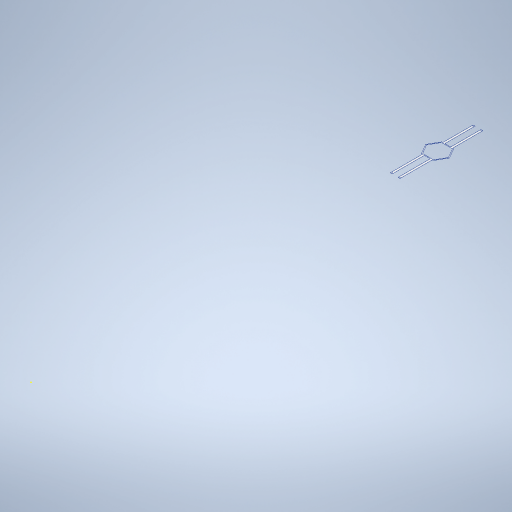
# Autodesk Inventor part: Suporte Drone
Saved by Autodesk Inventor 2024 (Build 280153000, 153)
## iProperties
Created: 2024-05-05
Part Number: Suporte Drone
Material: Alumínio 6061
Document SubType Name: Modeling
Designer: mathe
Density: 2.7 g/cm^3
Appearance: Alumínio - Plano
Author: mathe
Autodesk Inventor part; units mm, degrees
ref_plane "YZ Plane" through (0, 0, 0) normal (1, 0, 0) x (0, 1, 0)
ref_plane "XZ Plane" through (0, 0, 0) normal (0, 1, 0) x (-1, 0, 0)
ref_plane "XY Plane" through (0, 0, 0) normal (0, 0, 1) x (1, 0, 0)
sketch "Esboço1" plane through (0, 0, 0) normal (0, 1, 0) x (-1, 0, 0)
  circle A0 centre (4056.1731, -3688.1035) radius 2.5
  circle A1 centre (4056.1731, -4511.1035) radius 2.5
  circle A2 centre (3976.1731, -3688.1035) radius 2.5
  circle A3 centre (3976.1731, -4511.1035) radius 2.5
  line L0 (3904.5296, -4109.6035) -> (3960.3514, -4012.9174)
  line L1 (3960.3514, -4012.9174) -> (4071.9948, -4012.9174)
  line L2 (4071.9948, -4012.9174) -> (4127.8165, -4109.6035)
  line L3 (4127.8165, -4109.6035) -> (4071.9948, -4206.2895)
  line L4 (4071.9948, -4206.2895) -> (3960.3514, -4206.2895)
  line L5 (3960.3514, -4206.2895) -> (3904.5296, -4109.6035)
  line L6 (4136.5404, -4109.6035) -> (4076.3567, -4213.8446)
  line L7 (3955.9894, -4213.8446) -> (3895.8058, -4109.6035)
  line L8 (3895.8058, -4109.6035) -> (3955.9894, -4005.3623)
  line L9 (4076.3567, -4005.3623) -> (4136.5404, -4109.6035)
  line L10 (3986.1731, -3678.1035) -> (3986.1731, -4005.3623)
  line L11 (3986.1731, -4005.3623) -> (4046.1731, -4005.3623)
  line L12 (4046.1731, -4005.3623) -> (4046.1731, -3678.1035)
  line L13 (4046.1731, -4213.8446) -> (3986.1731, -4213.8446)
  line L14 (3986.1731, -4213.8446) -> (3986.1731, -4521.1035)
  line L15 (4046.1731, -4521.1035) -> (4046.1731, -4213.8446)
  line L16 (4066.1731, -3678.1035) -> (4046.1731, -3678.1035)
  line L17 (3986.1731, -3678.1035) -> (3966.1731, -3678.1035)
  line L18 (3966.1731, -4521.1035) -> (3986.1731, -4521.1035)
  line L19 (4046.1731, -4521.1035) -> (4066.1731, -4521.1035)
  line L20 (3966.1731, -4213.8446) -> (3955.9894, -4213.8446)
  line L21 (4076.3567, -4213.8446) -> (4066.1731, -4213.8446)
  line L22 (4046.1731, -4213.8446) -> (3986.1731, -4213.8446)
  line L23 (4066.1731, -4005.3623) -> (4076.3567, -4005.3623)
  line L24 (3955.9894, -4005.3623) -> (3966.1731, -4005.3623)
  line L25 (3986.1731, -4005.3623) -> (4046.1731, -4005.3623)
  line L26 (4066.1731, -4521.1035) -> (4066.1731, -4206.2895)
  line L27 (4066.1731, -4012.9174) -> (4066.1731, -3678.1035)
  line L28 (3966.1731, -3678.1035) -> (3966.1731, -4012.9174)
  line L29 (3966.1731, -4206.2895) -> (3966.1731, -4521.1035)
  point P0 (4016.1731, -4109.6035)
  point P1 (4016.1731, -4521.1035)
  point P2 (4016.1731, -4109.6035)
  dimension "d1" = 823
  dimension "d2" = 0
  dimension "d3" = 823
  dimension "d4" = 0
  dimension "d5" = 80
  dimension "d6" = 0
  dimension "d7" = 5
  dimension "d8" = 5
  dimension "d9" = 5
  dimension "d10" = 5
  dimension "d18" = 411.5
  dimension "d19" = 0
  dimension "d21" = 10
  dimension "d22" = 10
  constraints: 60 end point, 10 parallel, 9 point on line, 5 perpendicular, 4 centre point, 3 horizontal, 1 coincident, 22 other
  measures "d1" distance of A1.centre A0.centre
  measures "d2" horizontal distance of A1.centre A0.centre
  measures "d3" distance of A3.centre A2.centre
  measures "d4" horizontal distance of A3.centre A2.centre
  measures "d5" distance of A2.centre A0.centre
  measures "d6" vertical distance of A0.centre A2.centre
  measures "d7" diameter of A0
  measures "d8" diameter of A2
  measures "d9" diameter of A3
  measures "d10" diameter of A1
  measures "d18" distance of point (4016.173, -4521.103) point (4016.173, -4109.603)
  measures "d19" vertical distance of L2.end L0.start
  measures "d21" distance from line of L12 A0.centre
  measures "d22" distance from line of L10 A2.centre
extrude "Extrusão1" add sketch "Esboço1" along normal mid plane 0.3 contours L5 L4 L29 L20 L7 L8 L24 L28 L1 L0 | L28 L17 L10 L11 L12 L16 L27 L1 | L4 L26 L19 L15 L13 L14 L18 L29 | L27 L23 L9 L6 L21 L26 L4 L3 L2 L1
sketch "Esboço2" plane through (-4046.1731, 0.15, -3678.1035) normal (1, 0, 0) x (0, 0, -1)
  point P0 (-3678.1035, -0.15)
